Autodesk Fusion 360 part; units mm, degrees
note: some values were not read from the file. Set by a fixed rule: which sketch regions a step uses.
(part 2 of 2)
  line L227 (-18.8523, -1.1477) -> (-16.8879, -1.1477)
  line L228 (-16.8879, -1.1477) -> (-16.8879, -1.5384)
  spline S305 degree 2 poles (-16.8836, -3.7932) (-16.8836, -4.2416) (-17.174, -4.5384) knots 0 0 0 1 1 1
  spline S306 degree 2 poles (-17.174, -4.5384) (-17.4623, -4.8352) (-17.9, -4.8352) knots 0 0 0 1 1 1
  spline S307 degree 2 poles (-17.9, -4.8352) (-18.3249, -4.8352) (-18.6068, -4.5342) knots 0 0 0 1 1 1
  spline S308 degree 2 poles (-18.6068, -4.5342) (-18.8865, -4.2331) (-18.8865, -3.7762) knots 0 0 0 1 1 1
  spline S309 degree 2 poles (-18.8865, -3.7762) (-18.8865, -3.3342) (-18.6025, -3.0374) knots 0 0 0 1 1 1
  spline S310 degree 2 poles (-18.6025, -3.0374) (-18.3164, -2.7406) (-17.8893, -2.7406) knots 0 0 0 1 1 1
  spline S311 degree 2 poles (-17.8893, -2.7406) (-17.458, -2.7406) (-17.1719, -3.0395) knots 0 0 0 1 1 1
  spline S312 degree 2 poles (-17.1719, -3.0395) (-16.8836, -3.3406) (-16.8836, -3.7932) knots 0 0 0 1 1 1
  spline S313 degree 2 poles (-17.2338, -3.7719) (-17.2338, -3.4922) (-17.4174, -3.3128) knots 0 0 0 1 1 1
  spline S314 degree 2 poles (-17.4174, -3.3128) (-17.6011, -3.1335) (-17.885, -3.1335) knots 0 0 0 1 1 1
  spline S315 degree 2 poles (-17.885, -3.1335) (-18.1669, -3.1335) (-18.3463, -3.3171) knots 0 0 0 1 1 1
  spline S316 degree 2 poles (-18.3463, -3.3171) (-18.5235, -3.5007) (-18.5235, -3.789) knots 0 0 0 1 1 1
  spline S317 degree 2 poles (-18.5235, -3.789) (-18.5235, -4.0751) (-18.3441, -4.2566) knots 0 0 0 1 1 1
  spline S318 degree 2 poles (-18.3441, -4.2566) (-18.1626, -4.4402) (-17.8808, -4.4402) knots 0 0 0 1 1 1
  spline S319 degree 2 poles (-17.8808, -4.4402) (-17.6011, -4.4402) (-17.4174, -4.2502) knots 0 0 0 1 1 1
  spline S320 degree 2 poles (-17.4174, -4.2502) (-17.2338, -4.0601) (-17.2338, -3.7719) knots 0 0 0 1 1 1
  line L229 (-17.426, -6.8765) -> (-18.8523, -6.8765)
  line L230 (-18.8523, -6.8765) -> (-18.8523, -6.4858)
  line L231 (-18.8523, -6.4858) -> (-17.7591, -6.4858)
  spline S321 degree 2 poles (-17.7591, -6.4858) (-17.4324, -6.4858) (-17.3043, -6.3982) knots 0 0 0 1 1 1
  spline S322 degree 2 poles (-17.3043, -6.3982) (-17.174, -6.3107) (-17.174, -6.0929) knots 0 0 0 1 1 1
  spline S323 degree 2 poles (-17.174, -6.0929) (-17.174, -5.9712) (-17.2295, -5.8687) knots 0 0 0 1 1 1
  spline S324 degree 2 poles (-17.2295, -5.8687) (-17.285, -5.7683) (-17.426, -5.6381) knots 0 0 0 1 1 1
  line L232 (-17.426, -5.6381) -> (-18.8523, -5.6381)
  line L233 (-18.8523, -5.6381) -> (-18.8523, -5.2495)
  line L234 (-18.8523, -5.2495) -> (-16.8879, -5.2495)
  line L235 (-16.8879, -5.2495) -> (-16.8879, -5.6381)
  line L236 (-16.8879, -5.6381) -> (-17.1463, -5.6381)
  spline S325 degree 2 poles (-17.1463, -5.6381) (-16.8495, -5.9349) (-16.8495, -6.2189) knots 0 0 0 1 1 1
  spline S326 degree 2 poles (-16.8495, -6.2189) (-16.8495, -6.5925) (-17.2039, -6.7975) knots 0 0 0 1 1 1
  spline S327 degree 2 poles (-17.2039, -6.7975) (-16.8452, -7.1093) (-16.8452, -7.4488) knots 0 0 0 1 1 1
  spline S328 degree 2 poles (-16.8452, -7.4488) (-16.8452, -7.7349) (-17.0544, -7.9185) knots 0 0 0 1 1 1
  spline S329 degree 2 poles (-17.0544, -7.9185) (-17.2637, -8.1043) (-17.6929, -8.1043) knots 0 0 0 1 1 1
  line L237 (-17.6929, -8.1043) -> (-18.8523, -8.1043)
  line L238 (-18.8523, -8.1043) -> (-18.8523, -7.7157)
  line L239 (-18.8523, -7.7157) -> (-17.6886, -7.7157)
  spline S330 degree 2 poles (-17.6886, -7.7157) (-17.4431, -7.7157) (-17.3128, -7.6153) knots 0 0 0 1 1 1
  spline S331 degree 2 poles (-17.3128, -7.6153) (-17.1826, -7.5149) (-17.1826, -7.327) knots 0 0 0 1 1 1
  spline S332 degree 2 poles (-17.1826, -7.327) (-17.1826, -7.0858) (-17.426, -6.8765) knots 0 0 0 1 1 1
  line L240 (-17.9043, -10.3121) -> (-17.9043, -8.9306)
  spline S333 degree 2 poles (-17.9043, -8.9306) (-18.1861, -8.9456) (-18.3527, -9.1185) knots 0 0 0 1 1 1
  spline S334 degree 2 poles (-18.3527, -9.1185) (-18.5192, -9.2936) (-18.5192, -9.569) knots 0 0 0 1 1 1
  spline S335 degree 2 poles (-18.5192, -9.569) (-18.5192, -9.9534) (-18.2801, -10.2779) knots 0 0 0 1 1 1
  line L241 (-18.2801, -10.2779) -> (-18.6601, -10.2779)
  spline S336 degree 2 poles (-18.6601, -10.2779) (-18.7797, -10.0986) (-18.831, -9.9214) knots 0 0 0 1 1 1
  spline S337 degree 2 poles (-18.831, -9.9214) (-18.8822, -9.7463) (-18.8822, -9.5093) knots 0 0 0 1 1 1
  spline S338 degree 2 poles (-18.8822, -9.5093) (-18.8822, -9.1847) (-18.7477, -8.984) knots 0 0 0 1 1 1
  spline S339 degree 2 poles (-18.7477, -8.984) (-18.6132, -8.7833) (-18.3868, -8.6616) knots 0 0 0 1 1 1
  spline S340 degree 2 poles (-18.3868, -8.6616) (-18.1584, -8.542) (-17.8594, -8.542) knots 0 0 0 1 1 1
  spline S341 degree 2 poles (-17.8594, -8.542) (-17.411, -8.542) (-17.1313, -8.7961) knots 0 0 0 1 1 1
  spline S342 degree 2 poles (-17.1313, -8.7961) (-16.8495, -9.0502) (-16.8495, -9.4559) knots 0 0 0 1 1 1
  spline S343 degree 2 poles (-16.8495, -9.4559) (-16.8495, -9.8466) (-17.1228, -10.0794) knots 0 0 0 1 1 1
  spline S344 degree 2 poles (-17.1228, -10.0794) (-17.3961, -10.3121) (-17.8552, -10.3121) knots 0 0 0 1 1 1
  line L242 (-17.8552, -10.3121) -> (-17.9043, -10.3121)
  line L243 (-17.6715, -8.9391) -> (-17.6715, -9.9278)
  spline S345 degree 2 poles (-17.6715, -9.9278) (-17.4388, -9.9128) (-17.3128, -9.789) knots 0 0 0 1 1 1
  spline S346 degree 2 poles (-17.3128, -9.789) (-17.1868, -9.6651) (-17.1868, -9.4559) knots 0 0 0 1 1 1
  spline S347 degree 2 poles (-17.1868, -9.4559) (-17.1868, -9.2466) (-17.3128, -9.1121) knots 0 0 0 1 1 1
  spline S348 degree 2 poles (-17.3128, -9.1121) (-17.4388, -8.9797) (-17.6715, -8.9391) knots 0 0 0 1 1 1
  line L244 (-17.1996, -10.4573) -> (-16.4822, -11.1875)
  line L245 (-16.4822, -11.1875) -> (-16.8879, -11.1875)
  line L246 (-16.8879, -11.1875) -> (-16.8879, -11.8089)
  line L247 (-16.8879, -11.8089) -> (-17.2381, -11.8089)
  line L248 (-17.2381, -11.8089) -> (-17.2381, -11.1875)
  line L249 (-17.2381, -11.1875) -> (-18.2011, -11.1875)
  spline S349 degree 2 poles (-18.2011, -11.1875) (-18.5384, -11.1875) (-18.5384, -11.4673) knots 0 0 0 1 1 1
  spline S350 degree 2 poles (-18.5384, -11.4673) (-18.5384, -11.6765) (-18.3975, -11.9093) knots 0 0 0 1 1 1
  line L250 (-18.3975, -11.9093) -> (-18.7605, -11.9093)
  spline S351 degree 2 poles (-18.7605, -11.9093) (-18.8865, -11.6851) (-18.8865, -11.4203) knots 0 0 0 1 1 1
  spline S352 degree 2 poles (-18.8865, -11.4203) (-18.8865, -11.1534) (-18.7306, -10.9762) knots 0 0 0 1 1 1
  spline S353 degree 2 poles (-18.7306, -10.9762) (-18.6836, -10.9206) (-18.626, -10.8843) knots 0 0 0 1 1 1
  spline S354 degree 2 poles (-18.626, -10.8843) (-18.5662, -10.848) (-18.4722, -10.8224) knots 0 0 0 1 1 1
  spline S355 degree 2 poles (-18.4722, -10.8224) (-18.3761, -10.7989) (-18.1092, -10.7989) knots 0 0 0 1 1 1
  line L251 (-18.1092, -10.7989) -> (-17.2381, -10.7989)
  line L252 (-17.2381, -10.7989) -> (-17.2381, -10.4573)
  line L253 (-17.2381, -10.4573) -> (-17.1996, -10.4573)
  line L254 (-17.9043, -13.863) -> (-17.9043, -12.4815)
  spline S356 degree 2 poles (-17.9043, -12.4815) (-18.1861, -12.4964) (-18.3527, -12.6694) knots 0 0 0 1 1 1
  spline S357 degree 2 poles (-18.3527, -12.6694) (-18.5192, -12.8445) (-18.5192, -13.1199) knots 0 0 0 1 1 1
  spline S358 degree 2 poles (-18.5192, -13.1199) (-18.5192, -13.5043) (-18.2801, -13.8288) knots 0 0 0 1 1 1
  line L255 (-18.2801, -13.8288) -> (-18.6601, -13.8288)
  spline S359 degree 2 poles (-18.6601, -13.8288) (-18.7797, -13.6495) (-18.831, -13.4722) knots 0 0 0 1 1 1
  spline S360 degree 2 poles (-18.831, -13.4722) (-18.8822, -13.2972) (-18.8822, -13.0601) knots 0 0 0 1 1 1
  spline S361 degree 2 poles (-18.8822, -13.0601) (-18.8822, -12.7356) (-18.7477, -12.5349) knots 0 0 0 1 1 1
  spline S362 degree 2 poles (-18.7477, -12.5349) (-18.6132, -12.3342) (-18.3868, -12.2125) knots 0 0 0 1 1 1
  spline S363 degree 2 poles (-18.3868, -12.2125) (-18.1584, -12.0929) (-17.8594, -12.0929) knots 0 0 0 1 1 1
  spline S364 degree 2 poles (-17.8594, -12.0929) (-17.411, -12.0929) (-17.1313, -12.347) knots 0 0 0 1 1 1
  spline S365 degree 2 poles (-17.1313, -12.347) (-16.8495, -12.6011) (-16.8495, -13.0068) knots 0 0 0 1 1 1
  spline S366 degree 2 poles (-16.8495, -13.0068) (-16.8495, -13.3975) (-17.1228, -13.6302) knots 0 0 0 1 1 1
  spline S367 degree 2 poles (-17.1228, -13.6302) (-17.3961, -13.863) (-17.8552, -13.863) knots 0 0 0 1 1 1
  line L256 (-17.8552, -13.863) -> (-17.9043, -13.863)
  line L257 (-17.6715, -12.49) -> (-17.6715, -13.4786)
  spline S368 degree 2 poles (-17.6715, -13.4786) (-17.4388, -13.4637) (-17.3128, -13.3399) knots 0 0 0 1 1 1
  spline S369 degree 2 poles (-17.3128, -13.3399) (-17.1868, -13.216) (-17.1868, -13.0068) knots 0 0 0 1 1 1
  spline S370 degree 2 poles (-17.1868, -13.0068) (-17.1868, -12.7975) (-17.3128, -12.663) knots 0 0 0 1 1 1
  spline S371 degree 2 poles (-17.3128, -12.663) (-17.4388, -12.5306) (-17.6715, -12.49) knots 0 0 0 1 1 1
  line L258 (-16.8879, -14.7) -> (-17.3384, -14.7)
  line L259 (-17.3384, -14.7) -> (-17.3043, -14.7214)
  spline S372 degree 2 poles (-17.3043, -14.7214) (-16.8495, -15.0032) (-16.8495, -15.2851) knots 0 0 0 1 1 1
  spline S373 degree 2 poles (-16.8495, -15.2851) (-16.8495, -15.505) (-17.0715, -15.7441) knots 0 0 0 1 1 1
  line L260 (-17.0715, -15.7441) -> (-17.4132, -15.5391)
  spline S374 degree 2 poles (-17.4132, -15.5391) (-17.221, -15.3363) (-17.221, -15.1633) knots 0 0 0 1 1 1
  spline S375 degree 2 poles (-17.221, -15.1633) (-17.221, -14.9754) (-17.4003, -14.8367) knots 0 0 0 1 1 1
  spline S376 degree 2 poles (-17.4003, -14.8367) (-17.5797, -14.7) (-17.8253, -14.7) knots 0 0 0 1 1 1
  line L261 (-17.8253, -14.7) -> (-18.8523, -14.7)
  line L262 (-18.8523, -14.7) -> (-18.8523, -14.3093)
  line L263 (-18.8523, -14.3093) -> (-16.8879, -14.3093)
  line L264 (-16.8879, -14.3093) -> (-16.8879, -14.7)
  spline S377 degree 2 poles (-18.3761, -16.216) (-18.3761, -16.3249) (-18.4509, -16.4018) knots 0 0 0 1 1 1
  spline S378 degree 2 poles (-18.4509, -16.4018) (-18.5256, -16.4786) (-18.6345, -16.4786) knots 0 0 0 1 1 1
  spline S379 degree 2 poles (-18.6345, -16.4786) (-18.7413, -16.4786) (-18.8139, -16.4018) knots 0 0 0 1 1 1
  spline S380 degree 2 poles (-18.8139, -16.4018) (-18.8865, -16.327) (-18.8865, -16.216) knots 0 0 0 1 1 1
  spline S381 degree 2 poles (-18.8865, -16.216) (-18.8865, -16.1071) (-18.8139, -16.0324) knots 0 0 0 1 1 1
  spline S382 degree 2 poles (-18.8139, -16.0324) (-18.7413, -15.9577) (-18.6345, -15.9577) knots 0 0 0 1 1 1
  spline S383 degree 2 poles (-18.6345, -15.9577) (-18.5256, -15.9577) (-18.4509, -16.0324) knots 0 0 0 1 1 1
  spline S384 degree 2 poles (-18.4509, -16.0324) (-18.3761, -16.1071) (-18.3761, -16.216) knots 0 0 0 1 1 1
  line L265 (-18.3932, -18.4473) -> (-18.7776, -18.4473)
  spline S385 degree 2 poles (-18.7776, -18.4473) (-18.8865, -18.1548) (-18.8865, -17.8751) knots 0 0 0 1 1 1
  spline S386 degree 2 poles (-18.8865, -17.8751) (-18.8865, -17.4139) (-18.6132, -17.1384) knots 0 0 0 1 1 1
  spline S387 degree 2 poles (-18.6132, -17.1384) (-18.3398, -16.8651) (-17.8808, -16.8651) knots 0 0 0 1 1 1
  spline S388 degree 2 poles (-17.8808, -16.8651) (-17.4174, -16.8651) (-17.1334, -17.132) knots 0 0 0 1 1 1
  spline S389 degree 2 poles (-17.1334, -17.132) (-16.8495, -17.3989) (-16.8495, -17.8345) knots 0 0 0 1 1 1
  spline S390 degree 2 poles (-16.8495, -17.8345) (-16.8495, -17.9861) (-16.8794, -18.1057) knots 0 0 0 1 1 1
  spline S391 degree 2 poles (-16.8794, -18.1057) (-16.9071, -18.2274) (-16.9861, -18.4046) knots 0 0 0 1 1 1
  line L266 (-16.9861, -18.4046) -> (-17.4003, -18.4046)
  spline S392 degree 2 poles (-17.4003, -18.4046) (-17.2124, -18.11) (-17.2124, -17.858) knots 0 0 0 1 1 1
  spline S393 degree 2 poles (-17.2124, -17.858) (-17.2124, -17.5954) (-17.3982, -17.4267) knots 0 0 0 1 1 1
  spline S394 degree 2 poles (-17.3982, -17.4267) (-17.5818, -17.258) (-17.868, -17.258) knots 0 0 0 1 1 1
  spline S395 degree 2 poles (-17.868, -17.258) (-18.169, -17.258) (-18.3463, -17.4395) knots 0 0 0 1 1 1
  spline S396 degree 2 poles (-18.3463, -17.4395) (-18.5235, -17.6231) (-18.5235, -17.9327) knots 0 0 0 1 1 1
  spline S397 degree 2 poles (-18.5235, -17.9327) (-18.5235, -18.1569) (-18.3932, -18.4473) knots 0 0 0 1 1 1
  spline S398 degree 2 poles (-16.8836, -19.8288) (-16.8836, -20.2772) (-17.174, -20.574) knots 0 0 0 1 1 1
  spline S399 degree 2 poles (-17.174, -20.574) (-17.4623, -20.8708) (-17.9, -20.8708) knots 0 0 0 1 1 1
  spline S400 degree 2 poles (-17.9, -20.8708) (-18.3249, -20.8708) (-18.6068, -20.5697) knots 0 0 0 1 1 1
  spline S401 degree 2 poles (-18.6068, -20.5697) (-18.8865, -20.2687) (-18.8865, -19.8117) knots 0 0 0 1 1 1
  spline S402 degree 2 poles (-18.8865, -19.8117) (-18.8865, -19.3698) (-18.6025, -19.073) knots 0 0 0 1 1 1
  spline S403 degree 2 poles (-18.6025, -19.073) (-18.3164, -18.7762) (-17.8893, -18.7762) knots 0 0 0 1 1 1
  spline S404 degree 2 poles (-17.8893, -18.7762) (-17.458, -18.7762) (-17.1719, -19.0751) knots 0 0 0 1 1 1
  spline S405 degree 2 poles (-17.1719, -19.0751) (-16.8836, -19.3762) (-16.8836, -19.8288) knots 0 0 0 1 1 1
  spline S406 degree 2 poles (-17.2338, -19.8075) (-17.2338, -19.5278) (-17.4174, -19.3484) knots 0 0 0 1 1 1
  spline S407 degree 2 poles (-17.4174, -19.3484) (-17.6011, -19.169) (-17.885, -19.169) knots 0 0 0 1 1 1
  spline S408 degree 2 poles (-17.885, -19.169) (-18.1669, -19.169) (-18.3463, -19.3527) knots 0 0 0 1 1 1
  spline S409 degree 2 poles (-18.3463, -19.3527) (-18.5235, -19.5363) (-18.5235, -19.8246) knots 0 0 0 1 1 1
  spline S410 degree 2 poles (-18.5235, -19.8246) (-18.5235, -20.1107) (-18.3441, -20.2922) knots 0 0 0 1 1 1
  spline S411 degree 2 poles (-18.3441, -20.2922) (-18.1626, -20.4758) (-17.8808, -20.4758) knots 0 0 0 1 1 1
  spline S412 degree 2 poles (-17.8808, -20.4758) (-17.6011, -20.4758) (-17.4174, -20.2858) knots 0 0 0 1 1 1
  spline S413 degree 2 poles (-17.4174, -20.2858) (-17.2338, -20.0957) (-17.2338, -19.8075) knots 0 0 0 1 1 1
  spline S414 degree 2 poles (-18.3761, -21.5029) (-18.3761, -21.6117) (-18.4509, -21.6886) knots 0 0 0 1 1 1
  spline S415 degree 2 poles (-18.4509, -21.6886) (-18.5256, -21.7655) (-18.6345, -21.7655) knots 0 0 0 1 1 1
  spline S416 degree 2 poles (-18.6345, -21.7655) (-18.7413, -21.7655) (-18.8139, -21.6886) knots 0 0 0 1 1 1
  spline S417 degree 2 poles (-18.8139, -21.6886) (-18.8865, -21.6139) (-18.8865, -21.5029) knots 0 0 0 1 1 1
  spline S418 degree 2 poles (-18.8865, -21.5029) (-18.8865, -21.394) (-18.8139, -21.3192) knots 0 0 0 1 1 1
  spline S419 degree 2 poles (-18.8139, -21.3192) (-18.7413, -21.2445) (-18.6345, -21.2445) knots 0 0 0 1 1 1
  spline S420 degree 2 poles (-18.6345, -21.2445) (-18.5256, -21.2445) (-18.4509, -21.3192) knots 0 0 0 1 1 1
  spline S421 degree 2 poles (-18.4509, -21.3192) (-18.3761, -21.394) (-18.3761, -21.5029) knots 0 0 0 1 1 1
  line L267 (-18.8523, -23.5121) -> (-18.6025, -23.5121)
  spline S422 degree 2 poles (-18.6025, -23.5121) (-18.737, -23.3883) (-18.8117, -23.2281) knots 0 0 0 1 1 1
  spline S423 degree 2 poles (-18.8117, -23.2281) (-18.8865, -23.0701) (-18.8865, -22.9121) knots 0 0 0 1 1 1
  spline S424 degree 2 poles (-18.8865, -22.9121) (-18.8865, -22.7263) (-18.7947, -22.5683) knots 0 0 0 1 1 1
  spline S425 degree 2 poles (-18.7947, -22.5683) (-18.7007, -22.4125) (-18.5427, -22.3313) knots 0 0 0 1 1 1
  spline S426 degree 2 poles (-18.5427, -22.3313) (-18.3826, -22.2523) (-18.0132, -22.2523) knots 0 0 0 1 1 1
  line L268 (-18.0132, -22.2523) -> (-16.8879, -22.2523)
  line L269 (-16.8879, -22.2523) -> (-16.8879, -22.6409)
  line L270 (-16.8879, -22.6409) -> (-18.0089, -22.6409)
  spline S427 degree 2 poles (-18.0089, -22.6409) (-18.3185, -22.6409) (-18.4423, -22.7285) knots 0 0 0 1 1 1
  spline S428 degree 2 poles (-18.4423, -22.7285) (-18.564, -22.8182) (-18.564, -23.0402) knots 0 0 0 1 1 1
  spline S429 degree 2 poles (-18.564, -23.0402) (-18.564, -23.3178) (-18.2929, -23.5121) knots 0 0 0 1 1 1
  line L271 (-18.2929, -23.5121) -> (-16.8879, -23.5121)
  line L272 (-16.8879, -23.5121) -> (-16.8879, -23.9007)
  line L273 (-16.8879, -23.9007) -> (-18.8523, -23.9007)
  line L274 (-18.8523, -23.9007) -> (-18.8523, -23.5121)
  line L275 (-16.8879, -25.7242) -> (-16.8879, -26.1875)
  line L276 (-16.8879, -26.1875) -> (-17.8509, -25.3484)
  line L277 (-17.8509, -25.3484) -> (-18.8523, -26.3584)
  line L278 (-18.8523, -26.3584) -> (-18.8523, -25.8374)
  line L279 (-18.8523, -25.8374) -> (-17.8509, -24.853)
  line L280 (-17.8509, -24.853) -> (-16.8879, -25.7242)
  line L281 (-15.8694, -24.4473) -> (-15.8694, -24.8359)
  line L282 (-15.8694, -24.8359) -> (-18.8523, -24.8359)
  line L283 (-18.8523, -24.8359) -> (-18.8523, -24.4473)
  line L284 (-18.8523, -24.4473) -> (-15.8694, -24.4473)
extrude "Extrude4" cut sketch "Sketch5" against normal blind 0.1 contours L29 L30 L31 L32 L33 L34 L35 L36 L37 L38 L39 L40 L41 | S0 S1 S2 S3 S4 S5 S6 S7 | L42 L43 L44 L45 | L46 L47 S8 S9 S10 S11 L48 L49 L50 S12 S13 S14 S15 S16 S17 S18 S19 L51 L52 L53 | S20 S21 S22 S23 S24 S25 S26 S27 | L54 L55 L56 L57 | L58 S28 S29 S30 S31 S32 S33 S34 S35 S36 S37 S38 S39 L59 S40 S41 S42 S43 S44 S45 S46 S47 S48 S49 S50 | L60 L61 S51 S52 S53 S54 S55 S56 L62 L63 L64 | L65 S65 S66 S67 S68 S69 S70 S71 L66 S72 S73 S74 | L68 S78 S79 S80 S81 S82 S83 L69 S84 S85 S86 S87 S88 S89 S90 S91 | S92 S93 L70 L71 S94 S95 S96 L72 L73 L74 L75 L76 L77 L78 L79 L80 L81 L82 | L83 L84 S97 S98 S99 L85 S100 S101 S102 S103 L86 L87 L88 | S104 S105 S106 S107 S108 S109 S110 S111 | L89 L90 S120 S121 S122 S123 S124 S125 S126 L91 L92 L93 S127 S128 S129 S130 S131 S132 L94 L95 L96 S133 S134 S135 S136 S137 S138 L97 L98 L99 | L100 S139 S140 S141 S142 S143 S144 S145 L101 S146 S147 S148 | S152 S153 L103 L104 S154 S155 S156 L105 L106 L107 L108 L109 L110 L111 L112 L113 L114 L115 | L116 S157 S158 S159 S160 S161 S162 S163 L117 S164 S165 S166 | L119 L120 S170 S171 S172 L121 S173 S174 S175 S176 L122 L123 L124 | L125 S177 S178 S179 S180 S181 S182 L126 L127 L128 L129 L130 S183 S184 S185 S186 S187 S188 | L157 L158 L159 L160 L161 L162 L163 L164 L165 L166 L167 L168 L169 | L144 L145 L146 L147 L148 L149 L150 L151 L152 L153 L154 L155 L156 | L131 L132 L133 L134 L135 L136 L137 L138 L139 L140 L141 L142 L143 | S189 S190 S191 S192 S193 S194 S195 S196 | L170 L171 L172 S197 S198 S199 S200 L173 L174 L175 L176 L177 S201 S202 S203 S204 S205 L178 L179 L180 S206 S207 S208 | S209 S210 S211 S212 S213 S214 S215 S216 | L181 L182 L183 L184 | L185 S217 S218 S219 S220 L186 L187 L188 S221 S222 S223 L189 L190 L191 L192 | S224 S225 S226 S227 S228 S229 S230 S231 | L193 L194 L195 L196 | L197 S232 S233 S234 S235 S236 S237 S238 S239 S240 S241 S242 L198 S243 S244 S245 S246 S247 L199 S248 S249 S250 S251 S252 | L200 L201 S253 S254 S255 S256 S257 L202 L203 | L206 S264 S265 S266 L207 S267 S268 S269 S270 S271 S272 S273 S274 S275 L208 | L210 S280 S281 S282 S283 S284 S285 S286 L211 S287 S288 S289 S290 S291 S292 | L212 L213 L214 L215 L216 L217 S293 S294 L218 S295 S296 S297 S298 S299 L219 L220 L221 | L222 L223 S300 S301 L224 S302 S303 S304 L225 L226 L227 L228 | S305 S306 S307 S308 S309 S310 S311 S312 | L229 L230 L231 S321 S322 S323 S324 L232 L233 L234 L235 L236 S325 S326 S327 S328 S329 L237 L238 L239 S330 S331 S332 | L240 S333 S334 S335 L241 S336 S337 S338 S339 S340 S341 S342 S343 S344 L242 | L244 L245 L246 L247 L248 L249 S349 S350 L250 S351 S352 S353 S354 S355 L251 L252 L253 | L254 S356 S357 S358 L255 S359 S360 S361 S362 S363 S364 S365 S366 S367 L256 | L258 L259 S372 S373 L260 S374 S375 S376 L261 L262 L263 L264 | S377 S378 S379 S380 S381 S382 S383 S384 | L265 S385 S386 S387 S388 S389 S390 S391 L266 S392 S393 S394 S395 S396 S397 | S398 S399 S400 S401 S402 S403 S404 S405 | S414 S415 S416 S417 S418 S419 S420 S421 | L267 S422 S423 S424 S425 S426 L268 L269 L270 S427 S428 S429 L271 L272 L273 L274 | L275 L276 L277 L278 L279 L280 | L281 L282 L283 L284
